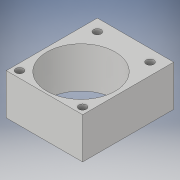
# Autodesk Inventor part: DPLX_P020_Camera Shroud Base_RevB
Saved by Autodesk Inventor 2018 (Build 220112000, 112)
## iProperties
Created: 2018-07-17
Part Number: DPLX_P020_Camera Shroud Base_RevB
Material: Generic
Document SubType Name: Modeling
Designer: DPLXuser
Density: 1 g/cm^3
Appearance: Default
Author: DPLXuser
Autodesk Inventor part; units mm, degrees
ref_plane "YZ Plane" through (0, 0, 0) normal (1, 0, 0) x (0, 1, 0)
ref_plane "XZ Plane" through (0, 0, 0) normal (0, 1, 0) x (-1, 0, 0)
ref_plane "XY Plane" through (0, 0, 0) normal (0, 0, 1) x (1, 0, 0)
sketch "Sketch3" plane through (0, 0, 0) normal (0, 1, 0) x (-1, 0, 0)
  line L0 (-17.78, -25.4) -> (17.78, -25.4)
  line L1 (17.78, -25.4) -> (17.78, 25.4)
  line L2 (17.78, 25.4) -> (-17.78, 25.4)
  line L3 (-17.78, 25.4) -> (-17.78, -25.4)
  line L4 (-17.78, -25.4) -> (17.78, 25.4) construction
  line L5 (17.78, -25.4) -> (-17.78, 25.4) construction
  point P0 (0, 0)
  dimension "d11" = 35.56
  dimension "d12" = 50.8
  constraints: 12 end point, 2 midpoint, 2 parallel, 1 horizontal, 1 perpendicular
  measures "d11" distance of L2.end L1.end
  measures "d12" distance of L1.end L0.end
extrude "Extrusion3" add sketch "Sketch3" along normal blind 19.05
sketch "Sketch4" plane through (0, 19.05, 0) normal (0, 1, 0) x (1, 0, 0)
  circle A0 centre (0, 0) radius 15.875
  dimension "d15" = 31.75
  constraints: 1 centre point, 1 coincident
  measures "d15" diameter of A0
extrude "Extrusion4" cut sketch "Sketch4" against normal blind 19.05
sketch "Sketch5" plane through (0, 19.05, 0) normal (0, 1, 0) x (1, 0, 0)
  line L0 (-17.6835, 25.5364) -> (55.9847, 25.5364) construction
  line L1 (-17.78, -25.4) -> (33.02, -25.4) construction
  circle A0 centre (12.2645, 19.8845) radius 1.778
  circle A1 centre (-12.2645, 19.8845) radius 1.778
  circle A2 centre (-12.2645, -19.8845) radius 1.778
  circle A3 centre (12.2645, -19.8845) radius 1.778
  point P0 (0, 0)
  point P1 (-17.78, 25.4)
  point P2 (17.78, -25.4)
  point P3 (17.78, 25.4)
  point P4 (0, 0)
  dimension "d20" = 3.556
  dimension "d21" = 3.556
  dimension "d22" = 3.556
  dimension "d23" = 3.556
  constraints: 4 centre point, 4 end point, 2 horizontal
  measures "d20" diameter of A0
  measures "d21" diameter of A1
  measures "d22" diameter of A2
  measures "d23" diameter of A3
extrude "Extrusion5" cut sketch "Sketch5" against normal blind 19.05
sketch "Sketch6" plane through (0, 19.05, 0) normal (0, 1, 0) x (1, 0, 0)
  line L0 (-17.78, -17.018) -> (17.78, -17.018)
  line L1 (-17.78, -17.018) -> (-17.78, -25.4)
  line L2 (-17.78, -25.4) -> (17.78, -25.4) projected
  line L3 (17.78, -25.4) -> (17.78, -17.018)
  point P0 (0, 0)
  point P1 (17.78, 25.4)
  point P2 (-17.78, 25.4)
  dimension "d26" = 42.418
  constraints: 6 end point, 1 vertical
  measures "d26" distance of point (-17.78, 25.4) L0.start
extrude "Extrusion6" cut sketch "Sketch6" against normal blind 19.05
sketch "Sketch7" plane through (0, 19.05, 0) normal (0, 1, 0) x (1, 0, 0)
  circle A0 centre (-14.6899, -13.9279) radius 1.778
  circle A1 centre (14.6899, -13.9279) radius 1.778
  point P0 (0, 0)
  point P1 (-17.78, -17.018)
  dimension "d30" = 3.556
  dimension "d31" = 3.556
  constraints: 2 centre point
  measures "d30" diameter of A0
  measures "d31" diameter of A1
extrude "Extrusion7" cut sketch "Sketch7" against normal blind 19.05
body "Solid2"
